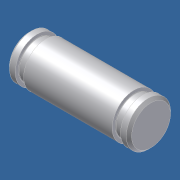
# Autodesk Inventor part: D-8381
Saved by Autodesk Inventor 2012 (Build 160160000, 160)
## iProperties
Category: PARTsolutions
Created: 2013-01-19
Part Number: D-8381
Catalog Web Link: www.cadenas.de
Description: Piston Rod Clevis for Original Line Cylinders - Pin -
Document SubType Name: Modeling
Designer: PARTsolutions
Material: Default
Density: 1 g/cm^3
NB: D-8381
NN: Piston Rod Clevis for Original Line Cylinders - Pin
NBSYN: $PN.
LINA: D-8381
PN: D-8381
L: 0.69000000
L1: 0.50000000
L2: 0.04750000
L4: 0.04750000
D: 0.25000000
D1: 0.21000000
CH: 0.01500000
R: 0.00250000
COLOR: 0.75,0.75,0.75,0.00
KT: DUMMY
SUPPLIER: Bimba
ARTICLENO: D-8381
BOMINFO: D-8381
CREATOR: CADENAS GmbH
PSOL_IDENT_0: {\\10.0.0.242\data_v9\23d-libs\bimba\bimba\bimba_imperial\bimba_full_line\original_line_cylinders\ac
PSOL_IDENT_1: cessories\piston_rod_clevis_pin.prj},199 {VTYP=3D},{NB=D-8381},{LINA=D-8381},{NN=Piston Rod Clevis f
PSOL_IDENT_2: or Original Line Cylinders - Pin},{DATE=06.12.2012 07:28:06},{GEOMDATE=06.12.2012 07:18:17},{VERSION
PSOL_IDENT_3: =},{LINEID=30},{LINESUBID=-1},{WBVAR=}  {NB=D-8381},{LINA=D-8381},{KT=DUMMY},{PN=D-8381},{L=0.690000
PSOL_IDENT_4: 00},{L1=0.50000000},{L2=0.04750000},{L4=0.04750000},{D=0.25000000},{D1=0.21000000},{CH=0.01500000},{
PSOL_IDENT_5: R=0.00250000},{COLOR=0.75,0.75,0.75,0.00}
Title: D-8381
Author: Cadenas PARTsolutions
Autodesk Inventor part; units mm, degrees
sketch "Sketch_1" plane through (0, 0, 0) normal (0, 0, 1) x (1, 0, 0)
  line L0 (8.763, 0) -> (-8.763, 0)
  line L1 (-8.763, 0) -> (-8.763, 2.794)
  line L2 (-8.763, 2.794) -> (-8.382, 3.175)
  line L3 (-8.382, 3.175) -> (-7.5565, 3.175)
  line L4 (-7.5565, 3.175) -> (-7.5565, 2.7305)
  arc A0 (-7.5565, 2.7305) -> (-7.493, 2.667) centre (-7.493, 2.7305) ccw
  line L5 (-7.493, 2.667) -> (-6.4135, 2.667)
  arc A1 (-6.4135, 2.667) -> (-6.35, 2.7305) centre (-6.4135, 2.7305) ccw
  line L6 (-6.35, 2.7305) -> (-6.35, 3.175)
  line L7 (-6.35, 3.175) -> (6.35, 3.175)
  line L8 (6.35, 3.175) -> (6.35, 2.7305)
  arc A2 (6.35, 2.7305) -> (6.4135, 2.667) centre (6.4135, 2.7305) ccw
  line L9 (6.4135, 2.667) -> (7.493, 2.667)
  arc A3 (7.493, 2.667) -> (7.5565, 2.7305) centre (7.493, 2.7305) ccw
  line L10 (7.5565, 2.7305) -> (7.5565, 3.175)
  line L11 (7.5565, 3.175) -> (8.382, 3.175)
  line L12 (8.382, 3.175) -> (8.763, 2.794)
  line L13 (8.763, 2.794) -> (8.763, 0)
  line L14 (8.763, 0) -> (-8.763, 0)
  constraints: 30 end point, 8 point on circle, 4 centre point
revolve "Revolution1" add sketch "Sketch_1" angle 360 about axis through (8.763, 0, 0) along (1, 0, 0)
ref_plane "pin_XY" through (0, 0, 0) normal (1, 0, 0) x (0, 0, -1)
ref_plane "pin_YZ" through (0, 0, 0) normal (0, 0, -1) x (0, 1, 0)
ref_plane "pin_ZX" through (0, 0, 0) normal (0, 1, 0) x (1, 0, 0)
ref_plane "rr1_XY" through (6.9532, 0, 0) normal (1, 0, 0) x (0, 0, -1)
ref_plane "rr1_YZ" through (6.9532, 0, 0) normal (0, 0, -1) x (0, 1, 0)
ref_plane "rr1_ZX" through (6.9532, 0, 0) normal (0, 1, 0) x (1, 0, 0)
ref_plane "rr2_XY" through (-6.9532, 0, 0) normal (1, 0, 0) x (0, 0, -1)
ref_plane "rr2_YZ" through (-6.9532, 0, 0) normal (0, 0, -1) x (0, 1, 0)
ref_plane "rr2_ZX" through (-6.9532, 0, 0) normal (0, 1, 0) x (1, 0, 0)
ref_plane "w21_XY" through (8.763, 0, 0) normal (0, 1, 0) x (1, 0, 0)
ref_plane "w21_YZ" through (8.763, 0, 0) normal (1, 0, 0) x (0, 0, -1)
ref_plane "w21_ZX" through (8.763, 0, 0) normal (0, 0, -1) x (0, 1, 0)
ref_plane "w22_XY" through (-8.763, 0, 0) normal (0, 1, 0) x (1, 0, 0)
ref_plane "w22_YZ" through (-8.763, 0, 0) normal (1, 0, 0) x (0, 0, -1)
ref_plane "w22_ZX" through (-8.763, 0, 0) normal (0, 0, -1) x (0, 1, 0)
ref_plane "p1_XY" through (0, 0, 3.175) normal (1, 0, 0) x (0, 0, -1)
ref_plane "p1_YZ" through (0, 0, 3.175) normal (0, 0, -1) x (0, 1, 0)
ref_plane "p1_ZX" through (0, 0, 3.175) normal (0, 1, 0) x (1, 0, 0)
ref_plane "p2_XY" through (0, 0, -3.175) normal (1, 0, 0) x (0, 0, -1)
ref_plane "p2_YZ" through (0, 0, -3.175) normal (0, 0, -1) x (0, 1, 0)
ref_plane "p2_ZX" through (0, 0, -3.175) normal (0, 1, 0) x (1, 0, 0)
body "Solid1"
